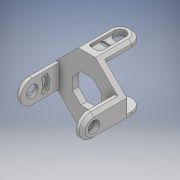
# Autodesk Inventor part: COXA2
Saved by Autodesk Inventor 2017.3 (Build 213256000, 256)
## iProperties
Created: 2017-09-24
Part Number: COXA2
Material: Generic
Document SubType Name: Modeling
Designer: Alexander Miller
Density: 1 g/cm^3
Appearance: Default
Author: Alexander Miller
Autodesk Inventor part; units mm, degrees
ref_plane "YZ Plane" through (0, 0, 0) normal (1, 0, 0) x (0, 1, 0)
ref_plane "XZ Plane" through (0, 0, 0) normal (0, 1, 0) x (-1, 0, 0)
ref_plane "XY Plane" through (0, 0, 0) normal (0, 0, 1) x (1, 0, 0)
sketch "Sketch1" plane through (0, 0, 0) normal (0, 1, 0) x (-1, 0, 0)
  line L0 (20, 7.5) -> (-20, 7.5) construction
  line L1 (-20, 7.5) -> (-20, -7.5)
  line L2 (-20, -7.5) -> (20, -7.5) construction
  line L3 (20, -7.5) -> (20, 7.5)
  line L4 (7.5, 20) -> (-7.5, 20)
  line L5 (-7.5, 20) -> (-7.5, -20) construction
  line L6 (-7.5, -20) -> (7.5, -20)
  line L7 (7.5, -20) -> (7.5, 20) construction
  line L8 (20, 7.5) -> (7.5, 20)
  line L9 (-7.5, 20) -> (-20, 7.5)
  line L10 (-20, -7.5) -> (-7.5, -20)
  line L11 (7.5, -20) -> (20, -7.5)
  point P0 (0, 0)
  point P1 (0, -7.5)
  point P2 (20, 0)
  point P3 (0, 20)
  point P4 (7.5, 0)
  dimension "d0" = 40
  dimension "d1" = 15
  constraints: 24 end point, 7 perpendicular, 4 midpoint, 4 parallel, 2 horizontal, 2 horizontal alignment, 2 vertical alignment
  measures "d0" distance of L1.end L2.end
  measures "d1" distance of L2.end L0.start
extrude "Extrusion1" add sketch "Sketch1" along normal blind 4
sketch "Sketch2" plane through (0, 0, 0) normal (0, -1, 0) x (1, 0, 0)
  line L0 (-20, 7.5) -> (-18, 7.5)
  line L1 (-18, 7.5) -> (-18, -7.5)
  line L2 (-18, -7.5) -> (-20, -7.5)
  line L3 (-20, -7.5) -> (-20, 7.5)
  line L4 (18, 7.5) -> (20, 7.5)
  line L5 (20, 7.5) -> (20, -7.5)
  line L6 (20, -7.5) -> (18, -7.5)
  line L7 (18, -7.5) -> (18, 7.5)
  line L8 (-20, 7.5) -> (-20, -7.5) projected
  line L9 (20, -7.5) -> (20, 7.5) projected
  point P0 (0, 0)
  point P1 (19, 7.5)
  point P2 (19, -7.5)
  point P3 (-19, -7.5)
  point P4 (-19, 7.5)
  dimension "d4" = 2
  constraints: 16 end point, 4 horizontal alignment, 4 midpoint, 4 parallel, 3 collinear, 2 horizontal, 2 perpendicular
  measures "d4" distance of L0.start L0.end
extrude "Extrusion2" add sketch "Sketch2" along normal blind 25
full round fillet "Fillet1" first side at (-19.3333, -8.3333, 7.5) centre faces at (-19.3333, -25, 2.5) second side at (-18.6667, -8.3333, -7.5)
full round fillet "Fillet2" first side at (19.3333, -8.3333, -7.5) centre faces at (19.3333, -25, 2.5) second side at (18.6667, -8.3333, 7.5)
sketch "Sketch3" plane through (0, 4, 0) normal (0, 1, 0) x (1, 0, 0)
  line L0 (-7.5, -20) -> (7.5, -20)
  line L1 (7.5, -20) -> (7.5, -18)
  line L2 (7.5, -18) -> (-7.5, -18)
  line L3 (-7.5, -18) -> (-7.5, -20)
  line L4 (-7.5, 18) -> (7.5, 18)
  line L5 (7.5, 18) -> (7.5, 20)
  line L6 (7.5, 20) -> (-7.5, 20)
  line L7 (-7.5, 20) -> (-7.5, 18)
  line L8 (-7.5, -20) -> (7.5, -20) projected
  line L9 (7.5, 20) -> (-7.5, 20) projected
  point P0 (0, 0)
  point P1 (-7.5, -19)
  point P2 (7.5, -19)
  point P3 (-7.5, 19)
  dimension "d7" = 2
  constraints: 16 end point, 4 parallel, 3 collinear, 3 midpoint, 3 vertical alignment, 2 horizontal, 2 perpendicular, 1 point on line
  measures "d7" distance of L2.end L0.start
extrude "Extrusion3" add sketch "Sketch3" along normal blind 25
full round fillet "Fillet3" first side at (7.5, 12.3333, 19.3333) centre faces at (2.5, 29, 19.3333) second side at (-7.5, 12.3333, 18.6667)
full round fillet "Fillet4" first side at (-7.5, 12.3333, -19.3333) centre faces at (2.5, 29, -18.6667) second side at (7.5, 12.3333, -18.6667)
sketch "Sketch4" plane through (20, 4, 7.5) normal (1, 0, 0) x (0, 0, -1)
  circle A0 centre (7.5, -21.5) radius 3.675
  arc A1 (0, -21.5) -> (15, -21.5) centre (7.5, -21.5) ccw projected
  point P0 (7.5, -4)
  dimension "d10" = 7.35
  constraints: 1 centre point, 1 concentric
  measures "d10" diameter of A0
extrude "Extrusion4" cut sketch "Sketch4" against normal up to surface (2 mm away)
sketch "Sketch5" plane through (7.5, 0, -20) normal (0, 0, -1) x (-1, 0, 0)
  circle A0 centre (7.5, 21.5) radius 3.675
  arc A1 (15, 21.5) -> (0, 21.5) centre (7.5, 21.5) ccw projected
  point P0 (7.5, 0)
  dimension "d13" = 7.35
  constraints: 1 centre point, 1 concentric
  measures "d13" diameter of A0
extrude "Extrusion5" cut sketch "Sketch5" against normal up to surface (2 mm away)
sketch "Sketch6" plane through (-20, 4, -7.5) normal (-1, 0, 0) x (0, 0, 1)
  circle A0 centre (7.5, -21.5) radius 3.75
  arc A1 (0, -21.5) -> (15, -21.5) centre (7.5, -21.5) ccw projected
  point P0 (7.5, -4)
  dimension "d16" = 7.5
  constraints: 1 centre point, 1 concentric
  measures "d16" diameter of A0
extrude "Extrusion6" cut sketch "Sketch6" against normal up to surface (2 mm away)
sketch "Sketch7" plane through (-7.5, 0, 20) normal (0, 0, 1) x (1, 0, 0)
  circle A0 centre (7.5, 21.5) radius 3.75
  arc A1 (15, 21.5) -> (0, 21.5) centre (7.5, 21.5) ccw projected
  point P0 (7.5, 0)
  dimension "d19" = 7.5
  constraints: 1 centre point, 1 concentric
  measures "d19" diameter of A0
extrude "Extrusion7" cut sketch "Sketch7" against normal up to surface (2 mm away)
sketch "Sketch13" plane through (-7.5, 0, 20) normal (0, 0, 1) x (1, 0, 0)
  line L0 (3.75, 21.5) -> (3.75, 4.5)
  line L1 (0, 4) -> (0, 21.5) projected
  line L2 (3.75, 4.5) -> (11.25, 4.5)
  circle A0 centre (7.5, 21.5) radius 3.75 projected
  arc A1 (15, 21.5) -> (0, 21.5) centre (7.5, 21.5) ccw projected
  line L3 (0, 4) -> (0, 21.5) projected
  line L4 (0, 0) -> (0, 4) projected
  line L5 (15, 0) -> (0, 0) projected
  line L6 (15, 0) -> (15, 4) projected
  line L7 (15, 4) -> (15, 21.5) projected
  circle A2 centre (7.5, 21.5) radius 3.75 projected
  line L8 (11.25, 4.5) -> (11.25, 21.5)
  arc A3 (11.25, 21.5) -> (3.75, 21.5) centre (7.5, 21.5) ccw
  point P0 (7.5, 0)
  point P1 (12, 0)
  point P2 (7.5, 4.5)
  dimension "d51" = 17
  constraints: 6 end point, 2 point on circle, 2 vertical, 1 centre point, 1 horizontal alignment, 1 midpoint, 1 parallel, 1 perpendicular, 1 vertical alignment, 2 other
  measures "d51" distance from line of L2 A1.centre
extrude "Extrusion13" add sketch "Sketch13" along normal blind 2
sketch "Sketch14" plane through (20, 4, 7.5) normal (1, 0, 0) x (0, 0, -1)
  circle A0 centre (7.5, -21.5) radius 3.675 projected
  arc A1 (0, -21.5) -> (15, -21.5) centre (7.5, -21.5) ccw projected
  line L0 (15, -4) -> (15, -21.5) projected
  line L1 (15, -4) -> (15, 0) projected
  line L2 (0, 0) -> (15, 0) projected
  line L3 (0, -4) -> (0, 0) projected
  line L4 (0, -4) -> (0, -21.5) projected
extrude "Extrusion14" add sketch "Sketch14" along normal blind 2
sketch "Sketch15" plane through (7.5, 0, -20) normal (0, 0, -1) x (-1, 0, 0)
  circle A0 centre (7.5, 21.5) radius 3.675 projected
  line L0 (0, 4) -> (0, 21.5) projected
  line L1 (0, 0) -> (0, 4) projected
  circle A1 centre (7.5, 21.5) radius 3.675 projected
  arc A2 (15, 21.5) -> (0, 21.5) centre (7.5, 21.5) ccw projected
  line L2 (0, 4) -> (0, 21.5) projected
  line L3 (0, 0) -> (0, 4) projected
  line L4 (15, 0) -> (0, 0) projected
  line L5 (15, 0) -> (15, 4) projected
  line L6 (15, 4) -> (15, 21.5) projected
extrude "Extrusion15" add sketch "Sketch15" along normal blind 2
sketch "Sketch16" plane through (-20, 4, -7.5) normal (-1, 0, 0) x (0, 0, 1)
  line L0 (11.25, -21.5) -> (11.25, -4.5)
  line L1 (11.25, -4.5) -> (3.75, -4.5)
  line L2 (3.75, -4.5) -> (3.75, -21.5)
  line L3 (0, -4) -> (0, -21.5) projected
  line L4 (0, 0) -> (15, 0) projected
  line L5 (15, -4) -> (15, -21.5) projected
  circle A0 centre (7.5, -21.5) radius 3.75 projected
  circle A1 centre (7.5, -21.5) radius 3.75 projected
  arc A2 (0, -21.5) -> (15, -21.5) centre (7.5, -21.5) ccw projected
  line L6 (15, -4) -> (15, -21.5) projected
  line L7 (15, -4) -> (15, 0) projected
  line L8 (0, 0) -> (15, 0) projected
  line L9 (0, -4) -> (0, 0) projected
  line L10 (0, -4) -> (0, -21.5) projected
  arc A3 (3.75, -21.5) -> (11.25, -21.5) centre (7.5, -21.5) ccw
  point P0 (7.5, -4)
  point P1 (7.5, -4.5)
  dimension "d60" = 17
  constraints: 6 end point, 2 perpendicular, 2 point on circle, 1 centre point, 1 horizontal alignment, 1 midpoint, 1 parallel, 1 vertical, 1 vertical alignment, 2 other
  measures "d60" distance of point (7.5, -4.5) point (7.5, -21.5)
extrude "Extrusion16" add sketch "Sketch16" along normal blind 2
chamfer "Chamfer5" distance 2 angle 45 12 edges at (-7.5, 10.75, -22) (0, 29, -22) (7.5, 10.75, -22) (-7.5, 10.75, 22) (0, 29, 22) (7.5, 10.75, 22) (-22, -6.75, 7.5) (-22, -25, 0) (-22, -6.75, -7.5) (22, -6.75, -7.5) (22, -25, 0) (22, -6.75, 7.5)
fillet "Fillet7" radius 1.75 4 edges at (3.75, 4.5, 21) (-3.75, 4.5, 21) (-21, -0.5, 3.75) (-21, -0.5, -3.75)
sketch "Sketch17" plane through (0, 4, 0) normal (0, 1, 0) x (1, 0, 0)
  line L0 (-9.4454, 3.9124) -> (-3.9124, 9.4454)
  line L1 (-3.9124, 9.4454) -> (3.9124, 9.4454)
  line L2 (3.9124, 9.4454) -> (9.4454, 3.9124)
  line L3 (9.4454, 3.9124) -> (9.4454, -3.9124)
  line L4 (9.4454, -3.9124) -> (3.9124, -9.4454)
  line L5 (3.9124, -9.4454) -> (-3.9124, -9.4454)
  line L6 (-3.9124, -9.4454) -> (-9.4454, -3.9124)
  line L7 (-9.4454, -3.9124) -> (-9.4454, 3.9124)
  line L8 (-7.5, -20) -> (-22, -5.5) projected
  point P0 (0, 0)
  point P1 (0, 0)
  dimension "d72" = 10
  constraints: 16 end point, 1 coincident, 17 other
  measures "d72" distance between parallel lines of L8 L6
extrude "Extrusion17" cut sketch "Sketch17" against normal through all
sketch "Sketch18" plane through (0, 21.5, 20) normal (0, 0, 1) x (1, 0, 0)
  circle A0 centre (0, 0) radius 3.75 projected
  arc A1 (-2.575, -8.6238) -> (2.575, -8.6238) centre (0, 0) ccw construction
  arc A2 (-2.9112, -9.7496) -> (2.9112, -9.7496) centre (0, 0) ccw
  arc A3 (-2.2388, -7.4979) -> (2.2388, -7.4979) centre (0, 0) ccw
  arc A4 (-2.2388, -7.4979) -> (-2.9112, -9.7496) centre (-2.575, -8.6238) ccw
  arc A5 (2.9112, -9.7496) -> (2.2388, -7.4979) centre (2.575, -8.6238) ccw
  line L0 (-3.75, 0) -> (-3.75, -15.25) projected
  point P0 (0, -21.5)
  point P1 (0, -9)
  dimension "d78" = 2.35
  dimension "d79" = 9
  constraints: 11 point on circle, 5 centre point, 5 tangent, 1 coincident, 1 horizontal alignment, 1 vertical alignment
  measures "d78" radial gap between concentric circles of A3 A2
  measures "d79" distance of point (0, -9) point (0, 0)
extrude "Extrusion18" cut sketch "Sketch18" against normal up to surface (2 mm away) contours A4 A3 A5 A2
sketch "Sketch19" plane through (7.5, 4, 18) normal (0, 0, -1) x (-1, 0, 0)
  circle A0 centre (7.5, 17.5) radius 3.75 projected
  arc A1 (3.8235, 9.2852) -> (11.1765, 9.2852) centre (7.5, 17.5) ccw construction
  arc A2 (2.935, 7.2999) -> (12.065, 7.2999) centre (7.5, 17.5) ccw
  arc A3 (4.712, 11.2704) -> (10.288, 11.2704) centre (7.5, 17.5) ccw
  arc A4 (4.712, 11.2704) -> (2.935, 7.2999) centre (3.8235, 9.2852) ccw
  arc A5 (12.065, 7.2999) -> (10.288, 11.2704) centre (11.1765, 9.2852) ccw
  arc A6 (10.4112, 7.7504) -> (9.7388, 10.0021) centre (10.075, 8.8762) ccw projected
  arc A7 (4.5888, 7.7504) -> (10.4112, 7.7504) centre (7.5, 17.5) ccw projected
  arc A8 (5.2612, 10.0021) -> (4.5888, 7.7504) centre (4.925, 8.8762) ccw projected
  arc A9 (5.2612, 10.0021) -> (9.7388, 10.0021) centre (7.5, 17.5) ccw projected
  circle A10 centre (7.5, 17.5) radius 3.75 projected
  arc A11 (15, 17.5) -> (0, 17.5) centre (7.5, 17.5) ccw projected
  line L0 (0, 0) -> (0, 17.5) projected
  line L1 (15, 0) -> (0, 0) projected
  line L2 (15, 0) -> (15, 17.5) projected
  point P0 (7.5, -4)
  point P1 (7.5, 8.5)
  dimension "d82" = 4.35
  constraints: 13 point on circle, 5 centre point, 4 tangent, 1 coincident, 1 vertical alignment
  measures "d82" radial gap between concentric circles of A2 A3
extrude "Extrusion19" cut sketch "Sketch19" against normal blind 1 contours A4 A3 A5 A2
sketch "Sketch20" plane through (-20, -17.5, 0) normal (-1, 0, 0) x (0, 0, 1)
  circle A0 centre (0, 0) radius 3.675 projected
  arc A1 (2.575, 8.6238) -> (-2.575, 8.6238) centre (0, 0) ccw construction
  arc A2 (2.9112, 9.7496) -> (-2.9112, 9.7496) centre (0, 0) ccw
  arc A3 (2.2388, 7.4979) -> (-2.2388, 7.4979) centre (0, 0) ccw
  arc A4 (2.2388, 7.4979) -> (2.9112, 9.7496) centre (2.575, 8.6238) ccw
  arc A5 (-2.9112, 9.7496) -> (-2.2388, 7.4979) centre (-2.575, 8.6238) ccw
  line L0 (-3.75, 15.25) -> (-3.75, 0) projected
  point P0 (0, 17.5)
  point P1 (0, 9)
  dimension "d85" = 2.35
  dimension "d86" = 9
  constraints: 11 point on circle, 5 centre point, 5 tangent, 1 coincident, 1 vertical alignment
  measures "d85" radial gap between concentric circles of A3 A2
  measures "d86" distance of point (0, 9) A0.centre
extrude "Extrusion20" cut sketch "Sketch20" against normal up to surface (2 mm away) contours A4 A3 A5 A2
sketch "Sketch21" plane through (-18, 0, 7.5) normal (1, 0, 0) x (0, 0, -1)
  arc A0 (4.5888, -7.7504) -> (5.2612, -10.0021) centre (4.925, -8.8762) ccw projected
  arc A1 (10.4112, -7.7504) -> (4.5888, -7.7504) centre (7.5, -17.5) ccw projected
  arc A2 (9.7388, -10.0021) -> (10.4112, -7.7504) centre (10.075, -8.8762) ccw projected
  arc A3 (9.7388, -10.0021) -> (5.2612, -10.0021) centre (7.5, -17.5) ccw projected
  circle A4 centre (7.5, -17.5) radius 3.75 projected
  arc A5 (0, -17.5) -> (15, -17.5) centre (7.5, -17.5) ccw projected
  line L0 (15, 0) -> (15, -17.5) projected
  line L1 (0, 0) -> (15, 0) projected
  line L2 (0, 0) -> (0, -17.5) projected
  arc A6 (11.1765, -9.2852) -> (3.8235, -9.2852) centre (7.5, -17.5) ccw construction
  arc A7 (12.065, -7.2999) -> (2.935, -7.2999) centre (7.5, -17.5) ccw
  arc A8 (10.288, -11.2704) -> (4.712, -11.2704) centre (7.5, -17.5) ccw
  arc A9 (10.288, -11.2704) -> (12.065, -7.2999) centre (11.1765, -9.2852) ccw
  arc A10 (2.935, -7.2999) -> (4.712, -11.2704) centre (3.8235, -9.2852) ccw
  point P0 (7.5, 0)
  point P1 (7.5, -8.5)
  dimension "d89" = 4.35
  constraints: 13 point on circle, 5 centre point, 4 tangent, 1 coincident, 1 vertical alignment
  measures "d89" radial gap between concentric circles of A7 A8
extrude "Extrusion21" cut sketch "Sketch21" against normal blind 1 contours A9 A8 A10 A7
sketch "Sketch22" plane through (-7.5, 4, -18) normal (0, 0, 1) x (1, 0, 0)
  circle A0 centre (7.5, 17.5) radius 3.675 projected
  circle A1 centre (7.5, 17.5) radius 2.675
  point P0 (7.5, -4)
  dimension "d93" = 1
  constraints: 1 centre point, 1 concentric
  measures "d93" radial gap between concentric circles of A0 A1
extrude "Extrusion22" add sketch "Sketch22" against normal blind 1
sketch "Sketch23" plane through (18, 0, -7.5) normal (-1, 0, 0) x (0, 0, 1)
  circle A0 centre (7.5, -17.5) radius 3.675 projected
  circle A1 centre (7.5, -17.5) radius 2.675
  point P0 (7.5, 0)
  dimension "d96" = 1
  constraints: 1 centre point, 1 concentric
  measures "d96" radial gap between concentric circles of A0 A1
extrude "Extrusion23" add sketch "Sketch23" against normal blind 1
equation "\"d10\" = bearing_A"
equation "\"d13\" = bearing_A"
equation "\"d16\" = servo_hat_A"
equation "\"d19\" = servo_hat_A"
equation "\"bearing_A\" = 7.35"
equation "\"servo_hat_A\" = 7.5"
body "Solid1"
